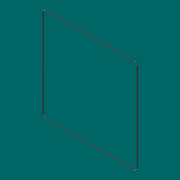
# Autodesk Inventor part: matingORing
Saved by Autodesk Inventor 2016 SP1 (Build 200210100, 210)
## iProperties
Created: 2016-04-01
Part Number: matingORing
Material: Rubber
Document SubType Name: Modeling
Designer: Sawaiz
Density: 0.93 g/cm^3
Appearance: Rubber - Black
Author: Sawaiz
Autodesk Inventor part; units mm, degrees
ref_plane "YZ Plane" through (0, 0, 0) normal (1, 0, 0) x (0, 1, 0)
ref_plane "XZ Plane" through (0, 0, 0) normal (0, 1, 0) x (-1, 0, 0)
ref_plane "XY Plane" through (0, 0, 0) normal (0, 0, 1) x (1, 0, 0)
sketch "Sketch1" plane through (0, 0, 0) normal (1, 0, 0) x (0, 1, 0)
  line L0 (-150, -150) -> (150, -150) construction
  line L1 (150, -150) -> (150, 150) construction
  line L2 (150, 150) -> (-150, 150) construction
  line L3 (-150, 150) -> (-150, -150) construction
  line L4 (-150, -150) -> (150, 150) construction
  line L5 (150, -150) -> (-150, 150) construction
  line L6 (-170, 170) -> (170, 170) construction
  line L7 (170, 170) -> (170, -170) construction
  line L8 (170, -170) -> (-170, -170) construction
  line L9 (-170, -170) -> (-170, 170) construction
  line L10 (174.7625, 174.7625) -> (-174.7625, 174.7625)
  line L11 (-174.7625, 174.7625) -> (-174.7625, -174.7625)
  line L12 (-174.7625, -174.7625) -> (174.7625, -174.7625)
  line L13 (174.7625, -174.7625) -> (174.7625, 174.7625)
  line L14 (-177.9375, 177.9375) -> (177.9375, 177.9375)
  line L15 (177.9375, 177.9375) -> (177.9375, -177.9375)
  line L16 (177.9375, -177.9375) -> (-177.9375, -177.9375)
  line L17 (-177.9375, -177.9375) -> (-177.9375, 177.9375)
  point P0 (0, 0)
  dimension "d0" = 300
  dimension "d1" = 300
  dimension "d2" = 20
  dimension "d3" = 4.7625
  dimension "d4" = 3.175
  constraints: 36 end point, 8 parallel, 4 perpendicular, 2 midpoint, 1 horizontal, 9 other
  measures "d0" distance of L2.end L1.end
  measures "d1" distance of L1.end L0.end
  measures "d2" distance between parallel lines of L2 L6
  measures "d3" distance between parallel lines of L6 L10
  measures "d4" distance between parallel lines of L10 L14
extrude "Extrusion1" add sketch "Sketch1" along normal blind 3.175
fillet "Fillet1" radius 7.9375 4 edges at (1.5875, 177.9375, 177.9375) (1.5875, -177.9375, 177.9375) (1.5875, -177.9375, -177.9375) (1.5875, 177.9375, -177.9375)
fillet "Fillet3" radius 4.7625 4 edges at (1.5875, 174.7625, -174.7625) (1.5875, -174.7625, 174.7625) (1.5875, 174.7625, 174.7625) (1.5875, -174.7625, -174.7625)
fillet "Fillet2" radius 1.5875 24 edges at (3.175, -175.6127, 175.6127) (3.175, -177.9375, 0) (3.175, -175.6127, -175.6127) (3.175, 0, -177.9375) (3.175, 175.6127, -175.6127) (3.175, 177.9375, 0) (3.175, 175.6127, 175.6127) (3.175, 0, 177.9375) (0, 175.6127, 175.6127) (0, 177.9375, 0) (0, 175.6127, -175.6127) (0, 0, -177.9375) (0, -175.6127, -175.6127) (0, -177.9375, 0) (0, -175.6127, 175.6127) (0, 0, 177.9375) (3.175, 174.7625, 0) (3.175, 0, -174.7625) (3.175, -174.7625, 0) (3.175, 0, 174.7625) (0, -174.7625, 0) (0, 0, -174.7625) (0, 174.7625, 0) (0, 0, 174.7625)
equation "\"d0\" = width"
equation "\"d1\" = height"
equation "\"d3\" = 0.375 * facingThickness"
equation "\"d4\" = 0.25 * facingThickness"
equation "\"d5\" = 0.25 * facingThickness"
equation "\"d7\" = 0.625 * facingThickness"
equation "\"d9\" = 0.375 * facingThickness"
equation "\"d8\" = 0.125 * facingThickness"
equation "\"width\" = 300"
equation "\"height\" = 300"
equation "\"facingThickness\" = 12.7"
equation "\"facingGasketThickness\" = 1.5875"
body "Solid1"
